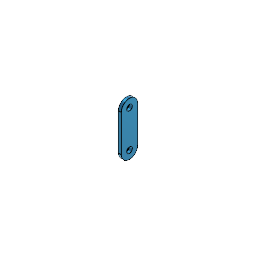
Bed Idler Support (Autodesk Fusion 360 design; units mm, degrees)
Autodesk Fusion 360 part; units mm, degrees
sketch "Sketch1" plane through (9.5, 0, 0) normal (1, 0, 0) x (0, 1, 0)
  circle A0 centre (26, 28) radius 2.75
  circle A1 centre (26, -8) radius 2.75
  line L0 (52, 20) -> (52, 0)
  line L1 (52, 0) -> (33.5, -16)
  line L2 (33.5, -16) -> (18.5, -16)
  line L3 (18.5, -16) -> (0, 0)
  line L4 (0, 0) -> (0, 20)
  line L5 (0, 20) -> (18.5, 36)
  line L6 (18.5, 36) -> (33.5, 36)
  line L7 (33.5, 36) -> (52, 20)
  circle A2 centre (44, 10) radius 2.75
  circle A3 centre (8, 10) radius 2.75
  circle A4 centre (26, 28) radius 8
  circle A5 centre (26, -8) radius 8
  line L8 (34, 28) -> (34, -8)
  line L9 (18, -8) -> (18, 28)
  dimension "d365" = 0
  dimension "d366" = 0
  dimension "d367" = 0
  dimension "d368" = 0
  dimension "d453" = 0
  dimension "d454" = 0
  dimension "d455" = 0
  dimension "d456" = 0
  dimension "d465" = 0
  dimension "d466" = 0
  dimension "d467" = 0
  dimension "d468" = 0
extrude "Extrude1" add sketch "Sketch1" along normal blind 3 contours A4 | A5 | A4 A5 L8 L9
named bodies: "Bed Idler Support"
